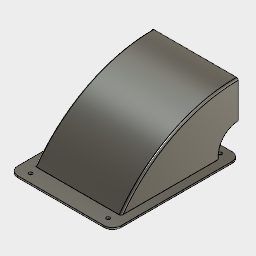
Outlet v6 (Autodesk Fusion 360 design; units mm, degrees)
Autodesk Fusion 360 part; units mm, degrees
note: some values were not read from the file. Chosen so that the rebuilt part matches the saved one: which pieces of a blend or face edit are solid. Set by a fixed rule: which sketch regions a step uses; which face or edge a step refers to.
sketch "Sketch3" plane through (0, 0, 0) normal (1, 0, 0) x (0, 1, 0) in component "Component"
  line L0 (0, 0) -> (0, -3.0821)
  line L1 (138.3345, 70.1394) -> (138.3532, 70.1394)
  line L2 (115, 3.5779) -> (115, 0)
  arc A0 (138.3345, 70.1394) -> (0, -3.0821) centre (138.3345, -97.1463) ccw
  line L3 (138.3532, 70.1394) -> (138.3439, 70.1394)
  line L4 (138.3439, 70.1394) -> (138.3439, 27.237)
  arc A1 (138.3439, 27.237) -> (115, 3.5779) centre (138.6612, 3.5779) ccw
  line L5 (0, 0) -> (115, 0)
extrude "Extrude1" add sketch "Sketch3" along normal blind 100 contours L1 L2 A0 L4 A1 L5 in component "Component"
shell "Shell1" thickness 2 removed faces 2 at (33.3333, 138.3439, 55.8386) at (33.3333, 39.7645, 0) in component "Component"
sketch "Sketch1" plane through (100, 0, 0) normal (1, 0, 0) x (0, 1, 0) in component "Component"
  line L0 (2.1467, 0) -> (115, 0)
  line L1 (115, 0) -> (115, 3.5779)
  arc A0 (138.3439, 27.237) -> (115, 3.5779) centre (138.6612, 3.5779) ccw
  line L2 (138.3439, 27.237) -> (138.3439, 70.1394)
  arc A1 (138.3345, 70.1394) -> (2.1467, 0) centre (138.3345, -97.1463) ccw
  line L3 (138.3439, 70.1394) -> (138.3345, 70.1394)
sketch "Sketch2" plane through (0, 0, 0) normal (0, 0, 1) x (1, 0, 0) in component "Component"
  line L0 (-10, -17.5633) -> (110, -17.5633)
  line L1 (110, -17.5633) -> (110, 131.1887)
  line L2 (110, 131.1887) -> (-10, 131.1887)
  line L3 (-10, 131.1887) -> (-10, -17.5633)
extrude "Extrude2" add sketch "Sketch2" against normal blind 2 in component "Component"
shell "Shell2" thickness 3 removed faces 2 at (30, 81.6047, -2) at (33.3333, -10.9933, 0) in component "Component"
hole "Hole3" at (95, -7.5633, 0) direction (0, 0, -1) diameter 4 depth 5 tip angle 118 in component "Component"
hole "Hole4" at (5, -7.5633, 0) direction (0, 0, -1) diameter 4 depth 5 tip angle 118 in component "Component"
hole "Hole5" at (95, 122.4367, 0) direction (0, 0, -1) diameter 4 depth 5 tip angle 118 in component "Component"
hole "Hole6" at (5, 122.4367, 0) direction (0, 0, -1) diameter 4 depth 5 tip angle 118 in component "Component"
fillet "Fillet1" radius 10 4 edges at (110, -17.5633, -1) (-10, -17.5633, -1) (-10, 131.1887, -1) (110, 131.1887, -1) in component "Component"
fillet "Fillet2" radius 2 4 edges at (100, 138.3392, 70.1394) (100, 61.7404, 51.5744) (0, 61.7404, 51.5744) (0, 138.3392, 70.1394) in component "Component"
component "Component" placed x (1, 0, 0) y (0, 1, 0) z (0, 0, 1) at (51.9773, -9.607, 8.5119)
